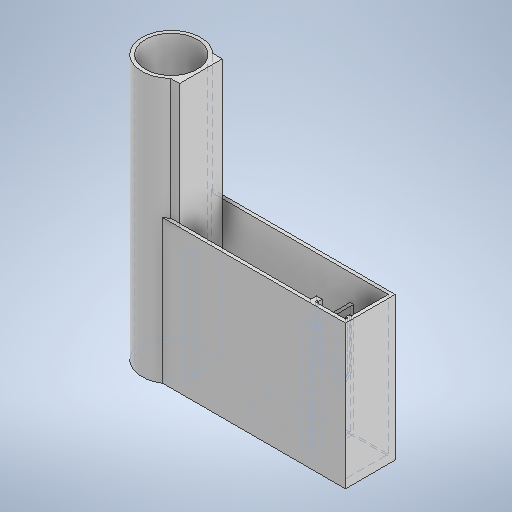
# Autodesk Inventor part: Open_source_chronograph_main_body_v2
Saved by Autodesk Inventor 2025 (Build 290162000, 162)
## iProperties
Created: 2025-03-27
Part Number: Open_source_chronograph_main_body_v2
Material: Generic
Document SubType Name: Modeling
Designer: Anarxus
Density: 1 g/cm^3
Appearance: Default
Author: Anarxus
Autodesk Inventor part; units mm, degrees
ref_plane "YZ Plane" through (0, 0, 0) normal (1, 0, 0) x (0, 1, 0)
ref_plane "XZ Plane" through (0, 0, 0) normal (0, 1, 0) x (-1, 0, 0)
ref_plane "XY Plane" through (0, 0, 0) normal (0, 0, 1) x (1, 0, 0)
sketch "Sketch1" plane through (0, 0, 0) normal (0, 1, 0) x (-1, 0, 0)
  circle A0 centre (0, 0) radius 15
  line L0 (-17, 0) -> (-91, 0)
  line L1 (-91, 0) -> (-115, 0)
  line L2 (-115, 0) -> (-115, -14.5)
  line L3 (-115, -14.5) -> (-8.8741, -14.5)
  line L4 (-0.35, 0) -> (-0.35, 13.2189)
  line L5 (-9.2718, 14.249) -> (-115, 14.249)
  line L6 (-115, 14.249) -> (-115, -14.5)
  line L7 (-113, -12.5) -> (-11.5217, -12.5)
  line L8 (-113, -12.5) -> (-113, 12.249)
  line L9 (-113, 12.249) -> (-11.7882, 12.249)
  circle A1 centre (0, 0) radius 17
  line L10 (-17, 0) -> (-17, 12.249)
  line L11 (-17, 0) -> (-17, -12.5)
  line L12 (-91, -12.5) -> (-91, 12.249)
  line L13 (-93, -12.5) -> (-93, 12.249)
  line L14 (-17, 12.249) -> (-17, 9.249)
  line L15 (-17, 9.249) -> (-20, 9.249)
  line L16 (-20, 9.249) -> (-20, 12.249)
  line L17 (-20, 12.249) -> (-17, 12.249)
  line L18 (-17, 12.249) -> (-17, 9.249)
  line L19 (-91, 9.249) -> (-88, 9.249)
  line L20 (-88, 9.249) -> (-88, 12.249)
  line L21 (-88, 12.249) -> (-91, 12.249)
  line L22 (-91, 12.249) -> (-91, 9.249)
  line L23 (-17, 9.249) -> (-17, 7.549)
  line L24 (-17, 7.549) -> (-20, 7.549)
  line L25 (-20, 7.549) -> (-20, 4.2225)
  line L26 (-20, 4.2225) -> (-17, 4.2225)
  line L27 (-17, 4.2225) -> (-17, 7.549)
  line L28 (-91, 7.549) -> (-88, 7.549)
  line L29 (-88, 7.549) -> (-88, 4.9725)
  line L30 (-88, 4.9725) -> (-91, 4.9725)
  line L31 (-91, 4.9725) -> (-91, 7.549)
  line L32 (-17, 7.549) -> (-20, 7.549)
  line L33 (-20, 7.549) -> (-20, 9.249)
  line L34 (-20, 9.249) -> (-17, 9.249)
  line L35 (-17, 9.249) -> (-17, 7.549)
  line L36 (-91, 7.549) -> (-88, 7.549)
  line L37 (-88, 7.549) -> (-88, 9.249)
  line L38 (-88, 9.249) -> (-91, 9.249)
  line L39 (-91, 9.249) -> (-91, 7.549)
  line L40 (-91, 7.549) -> (-70.5, 7.549)
  line L41 (-70.5, 7.549) -> (-70.5, 3.549)
  line L42 (-70.5, 3.549) -> (-47.5, 3.549)
  line L43 (-47.5, 3.549) -> (-47.5, -9.451)
  line L44 (-47.5, -9.451) -> (-70.5, -9.451)
  line L45 (-70.5, -9.451) -> (-70.5, 3.549)
  point P0 (-93, 12.249)
  dimension "d0" = 30
  dimension "d1" = 74
  dimension "d2" = 24
  dimension "d3" = 14.5
  dimension "d4" = 29
  dimension "d5" = 2
  dimension "d6" = 2
  dimension "d7" = 2
  dimension "d9" = 2
  dimension "d10" = 3
  dimension "d11" = 3
  dimension "d12" = 3
  dimension "d13" = 1.7
  dimension "d14" = 3
  dimension "d15" = 3
  dimension "d16" = 20.5
  dimension "d17" = 4
  dimension "d18" = 23
  dimension "d19" = 13
  constraints: 92 end point, 18 parallel, 15 point on line, 10 horizontal, 10 perpendicular, 5 point on circle, 2 centre point, 2 vertical, 1 coincident
  measures "d0" diameter of A0
  measures "d1" distance of L0.start L0.end
  measures "d2" distance of L0.end L1.end
  measures "d3" distance of L1.end L2.end
  measures "d4" distance of L4.end L3.end
  measures "d5" distance between parallel lines of L3 L7
  measures "d6" distance between parallel lines of L6 L8
  measures "d7" radial gap between concentric circles of A0 A1
  measures "d9" distance between parallel lines of L12 L13
  measures "d10" distance of L10.end L14.end
  measures "d11" distance of L16.end L17.end
  measures "d12" distance of L21.end L20.end
  measures "d13" distance of L14.end L23.end
  measures "d14" distance of L26.end L25.end
  measures "d15" distance of L29.end L30.end
  measures "d16" distance of L28.start L40.end
  measures "d17" distance of L40.end L41.end
  measures "d18" distance of L43.end L44.end
  measures "d19" distance of L42.end L43.end
extrude "Extrusion1" add sketch "Sketch1" against normal blind 3 contours L11 L7 L12 L0 L45 L44 L43 | L10 L9 A1 | A1 | L0 L43 L42 L41 L40 L37 L20 L9 L16 L33 L25 L26 L10 | A1 L7 L11 | L9 L8 L1 L6 L5 A1 | A1 L3 L2 L1 L8 L7 | L26 L25 L24 L10 | L0 L12 L30 L29 L40 L41 L45 | L10 L15 L16 L9 | L24 L33 L15 L10 | L7 L13 L1 L12 | L1 L13 L9 L12 | L7 L8 L1 L13 | L1 L8 L9 L13 | L12 L28 L29 L30 | L20 L19 L12 L9 | L12 L19 L37 L28
extrude "Extrusion2" add sketch "Sketch1" along normal blind 150 contours A1
extrude "Extrusion3" add sketch "Sketch1" along normal blind 150 contours L10 L9 A1 | A1 L7 L11
extrude "Extrusion4" add sketch "Sketch1" along normal blind 80 contours L9 L8 L1 L6 L5 A1 | A1 L3 L2 L1 L8 L7
extrude "Extrusion5" add sketch "Sketch1" along normal blind 3 contours L24 L33 L15 L10 | L12 L19 L37 L28
extrude "Extrusion6" add sketch "Sketch1" along normal blind 65 contours L26 L25 L24 L10 | L10 L15 L16 L9 | L7 L13 L1 L12 | L1 L13 L9 L12 | L12 L28 L29 L30 | L20 L19 L12 L9
sketch "Sketch2" plane through (0, 65, 0) normal (0, 1, 0) x (1, 0, 0)
  line L0 (113, -12.249) -> (113, 12.5) projected
  line L1 (113, -12.249) -> (113, -10.999)
  line L2 (113, -10.999) -> (112, -10.999)
  line L3 (112, -10.999) -> (112, -8.999)
  line L4 (112, -8.999) -> (113, -8.999)
  line L5 (113, -12.249) -> (95.4, -12.249)
  line L6 (113, -12.249) -> (17, -12.249) projected
  line L7 (95.4, -12.249) -> (95.4, -10.999)
  line L8 (95.4, -10.999) -> (96.4, -10.999)
  line L9 (96.4, -10.999) -> (96.4, -8.9987)
  line L10 (96.4, -8.9987) -> (93, -8.9987)
  line L11 (93, -12.249) -> (93, 12.5) projected
  line L12 (93, -8.9987) -> (93, -12.249)
  line L13 (93, -12.249) -> (95.4, -12.249)
  point P0 (0, 0)
  dimension "d32" = 1.25
  dimension "d33" = 1
  dimension "d34" = 2
  dimension "d35" = 17.6
  dimension "d36" = 1
  constraints: 22 end point, 6 perpendicular, 3 point on line, 1 collinear, 1 horizontal, 1 vertical
  measures "d32" distance of L0.start L1.end
  measures "d33" distance of L1.end L2.end
  measures "d34" distance of L2.end L3.end
  measures "d35" distance of L0.start L5.end
  measures "d36" distance of L7.end L8.end
extrude "Extrusion7" add sketch "Sketch2" along normal up to surface (15 mm away)
extrude "Extrusion8" add sketch "Sketch2" against normal blind 13.5
sketch "Sketch3" plane through (93, 0, -12.5) normal (1, 0, 0) x (0, 0, -1)
  line L0 (-23.499, 51.5) -> (-24.749, 51.5) projected
  line L1 (-24.749, 51.5) -> (-21.4987, 51.5)
  line L2 (-24.749, 51.5) -> (-21.4987, 51.5)
  line L3 (-24.749, 51.5) -> (-24.749, 48.25)
  line L4 (-24.749, 48.25) -> (-21.4987, 51.5)
  point P0 (-12.5, 0)
  dimension "d44" = 3.25
  constraints: 8 end point, 1 collinear, 1 horizontal, 1 perpendicular
  measures "d44" distance of L0.end L3.end
extrude "Extrusion9" add sketch "Sketch3" along normal up to surface (20 mm away)
sketch "Sketch4" plane through (95.4, 51.5, 12.249) normal (0, 1, 0) x (1, 0, 0)
  line L0 (1, 3.2503) -> (1, 1.25) projected
  line L1 (17.6, 1.25) -> (16.6, 1.25) projected
  line L2 (1, 3.2503) -> (16.6, 3.2503)
  line L3 (16.6, 3.2503) -> (16.6, 1.25)
  line L4 (16.6, 1.25) -> (1, 1.25)
  line L5 (1, 1.25) -> (1, 3.2503)
  point P0 (-95.4, 12.249)
  constraints: 8 end point, 2 parallel, 1 horizontal, 1 perpendicular
extrude "Extrusion10" cut sketch "Sketch4" against normal blind 10
sketch "Sketch5" plane through (17, 80, -12.5) normal (0, 0, 1) x (1, 0, 0)
  line L0 (74, -77) -> (71, -77) projected
  line L1 (74, -77) -> (74, -61)
  line L2 (74, -80) -> (74, -15) projected
  line L3 (74, -61) -> (65, -61)
  circle A0 centre (65, -61) radius 3.1
  line L4 (65, -61) -> (65, -49.5)
  line L5 (65, -49.5) -> (65, -38)
  circle A1 centre (65, -49.5) radius 3.1
  circle A2 centre (65, -38) radius 3.1
  circle A3 centre (65, -38) radius 5.1
  circle A4 centre (65, -49.5) radius 5.1
  circle A5 centre (65, -61) radius 5.1
  line L6 (3, -80) -> (71, -80) projected
  line L7 (64, -80) -> (66, -80)
  line L8 (66, -31.3579) -> (64, -31.3579)
  line L9 (64, -43.001) -> (64, -44.499)
  line L10 (66, -44.499) -> (66, -43.001)
  line L11 (66, -55.999) -> (66, -54.501)
  line L12 (64, -54.501) -> (64, -55.999)
  line L13 (64, -66.001) -> (64, -80)
  line L14 (66, -80) -> (66, -66.001)
  point P0 (-17, -80)
  dimension "d47" = 16
  dimension "d48" = 9
  dimension "d49" = 6.2
  dimension "d50" = 11.5
  dimension "d51" = 11.5
  dimension "d52" = 6.2
  dimension "d53" = 6.2
  dimension "d54" = 2
  dimension "d55" = 2
  dimension "d56" = 2
  dimension "d57" = 2
  constraints: 24 end point, 10 parallel, 10 point on circle, 6 centre point, 4 perpendicular, 3 coincident, 3 point on line, 1 horizontal, 1 vertical
  measures "d47" distance of L0.start L1.end
  measures "d48" distance of L1.end L3.end
  measures "d49" diameter of A0
  measures "d50" distance of L4.start L4.end
  measures "d51" distance of L4.end L5.end
  measures "d52" diameter of A1
  measures "d53" diameter of A2
  measures "d54" radial gap between concentric circles of A2 A3
  measures "d55" radial gap between concentric circles of A1 A4
  measures "d56" radial gap between concentric circles of A0 A5
  measures "d57" distance of L8.end L8.start
extrude "Extrusion11" cut sketch "Sketch5" against normal blind 10 contours A0 L4 L3 | L3 L4 A0 | A1 L5 L4 | L4 L5 A1 | A2
body "Solid1"
